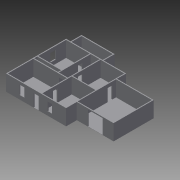
# Autodesk Inventor part: 305 Manning
Saved by Autodesk Inventor 2013 SP2 (Build 170200200, 200)
## iProperties
Created: 2014-06-03
Part Number: 305 Manning
Material: Generic
Document SubType Name: Modeling
Designer: jmw3
Density: 1 g/cm^3
Author: jmw3
Autodesk Inventor part; units mm, degrees
ref_plane "YZ Plane" through (0, 0, 0) normal (1, 0, 0) x (0, 1, 0)
ref_plane "XZ Plane" through (0, 0, 0) normal (0, 1, 0) x (-1, 0, 0)
ref_plane "XY Plane" through (0, 0, 0) normal (0, 0, 1) x (1, 0, 0)
sketch "Sketch1" plane through (0, 0, 0) normal (0, 1, 0) x (-1, 0, 0)
  line L0 (4978.4, 4978.4) -> (4978.4, -4978.4)
  line L1 (8188.96, 0) -> (-14284.96, 0) projected
  line L2 (0, -9164.32) -> (0, 7335.52) projected
  line L3 (-4978.4, -3454.4) -> (-11074.4, -3454.4)
  line L4 (-11074.4, -3454.4) -> (-11074.4, 3200.4)
  line L5 (-4978.4, -3302) -> (-10922, -3302)
  line L6 (-10922, -3302) -> (-10922, 3048)
  line L7 (4089.4, -4978.4) -> (-1092.2, -4978.4)
  line L8 (-1244.6, -4978.4) -> (-1244.6, -6807.2)
  line L9 (-1244.6, -6807.2) -> (4241.8, -6807.2)
  line L10 (4241.8, -6807.2) -> (4241.8, -4978.4)
  line L11 (4089.4, -6654.8) -> (-1092.2, -6654.8)
  line L12 (-1092.2, -6654.8) -> (-1092.2, -4978.4)
  line L13 (-1092.2, -4978.4) -> (4089.4, -4978.4)
  line L14 (4089.4, -4978.4) -> (4089.4, -6654.8)
  line L15 (-1244.6, -4978.4) -> (-4978.4, -4978.4)
  line L16 (4978.4, -4978.4) -> (4241.8, -4978.4)
  line L17 (4089.4, -4978.4) -> (-1092.2, -4978.4)
  line L18 (-4978.4, -4978.4) -> (-4978.4, -3454.4)
  line L19 (-4978.4, 3200.4) -> (-4978.4, 4978.4)
  line L20 (-6807.2, 3048) -> (-6807.2, 3200.4)
  line L21 (-9245.6, 3048) -> (-9245.6, 3200.4)
  line L22 (-10922, 3048) -> (-9245.6, 3048)
  line L23 (-6807.2, 3048) -> (-4978.4, 3048)
  line L24 (-11074.4, 3200.4) -> (-9245.6, 3200.4)
  line L25 (-6807.2, 3200.4) -> (-4978.4, 3200.4)
  line L26 (-406.4, 4826) -> (-406.4, 4978.4)
  line L27 (406.4, 4826) -> (406.4, 4978.4)
  line L28 (-4978.4, 4978.4) -> (-406.4, 4978.4)
  line L29 (406.4, 4978.4) -> (4978.4, 4978.4)
  line L30 (406.4, 4826) -> (4826, 4826)
  line L31 (4826, -203.2) -> (889, -203.2)
  line L32 (4826, -50.8) -> (889, -50.8)
  line L33 (-4826, -203.2) -> (-889, -203.2)
  line L34 (-4826, -50.8) -> (-889, -50.8)
  line L35 (-4826, -1905) -> (-4978.4, -1905)
  line L36 (-4826, -2692.4) -> (-4978.4, -2692.4)
  line L37 (-4978.4, 3048) -> (-4978.4, -1905)
  line L38 (-4978.4, -2692.4) -> (-4978.4, -3302)
  line L39 (-4978.4, 3048) -> (-4978.4, -1905)
  line L40 (-4978.4, -2692.4) -> (-4978.4, -3302)
  line L41 (-4826, -4826) -> (-4826, -2692.4)
  line L42 (-4978.4, -3302) -> (-4978.4, -2692.4)
  line L43 (-4978.4, -1905) -> (-4978.4, 3048)
  line L44 (-4826, -1905) -> (-4826, -203.2)
  line L45 (-4826, -50.8) -> (-4826, 4826)
  line L46 (-4826, 4826) -> (-889, 4826)
  line L47 (-736.6, 4826) -> (-406.4, 4826)
  line L48 (4826, -203.2) -> (4826, -4826)
  line L49 (4826, -4826) -> (889, -4826)
  line L50 (736.6, -4826) -> (-736.6, -4826)
  line L51 (-889, -4826) -> (-4826, -4826)
  line L52 (889, -2692.4) -> (736.6, -2692.4)
  line L53 (889, -3454.4) -> (736.6, -3454.4)
  line L54 (-736.6, -1016) -> (-889, -1016)
  line L55 (-736.6, -1828.8) -> (-889, -1828.8)
  line L56 (-254, 457.2) -> (-254, 609.6)
  line L57 (558.8, 609.6) -> (4826, 609.6)
  line L58 (736.6, -50.8) -> (736.6, 457.2)
  line L59 (889, -50.8) -> (889, 457.2)
  line L60 (-736.6, 3048) -> (-889, 3048)
  line L61 (-736.6, 2286) -> (-889, 2286)
  line L62 (558.8, 457.2) -> (558.8, 609.6)
  line L63 (-254, 609.6) -> (-736.6, 609.6)
  line L64 (-736.6, 457.2) -> (-254, 457.2)
  line L65 (-736.6, -50.8) -> (-736.6, 457.2)
  line L66 (4826, 457.2) -> (889, 457.2)
  line L67 (736.6, 457.2) -> (558.8, 457.2)
  line L68 (-736.6, 609.6) -> (-736.6, 2286)
  line L69 (-736.6, 3048) -> (-736.6, 4826)
  line L70 (-889, -50.8) -> (-889, 2286)
  line L71 (-889, 3048) -> (-889, 4826)
  line L72 (-736.6, -50.8) -> (-736.6, -1016)
  line L73 (-736.6, -1828.8) -> (-736.6, -4826)
  line L74 (-889, -203.2) -> (-889, -1016)
  line L75 (-889, -1828.8) -> (-889, -4826)
  line L76 (736.6, -50.8) -> (736.6, -2692.4)
  line L77 (736.6, -3454.4) -> (736.6, -4826)
  line L78 (889, -203.2) -> (889, -2692.4)
  line L79 (889, -3454.4) -> (889, -4826)
  line L80 (4826, 4826) -> (4826, 609.6)
  line L81 (4826, 457.2) -> (4826, -50.8)
  point P0 (0, 0)
  dimension "d8" = 152.4
  dimension "d9" = 152.4
  dimension "d12" = 736.6
  dimension "d14" = 152.4
  dimension "d15" = 152.4
  dimension "d16" = 152.4
  dimension "d17" = 1828.8
  dimension "d19" = 1524
  dimension "d22" = 9956.8
  dimension "d23" = 3733.8
  dimension "d24" = 1828.8
  dimension "d25" = 1828.8
  dimension "d26" = 6654.8
  dimension "d27" = 152.4
  dimension "d28" = 4572
  dimension "d29" = 812.8
  dimension "d30" = 9956.8
  dimension "d32" = 152.4
  dimension "d35" = 1701.8
  dimension "d36" = 2489.2
  dimension "d38" = 5486.4
  dimension "d40" = 152.4
  dimension "d41" = 4622.8
  dimension "d42" = 152.4
  dimension "d43" = 6096
  dimension "d44" = 2489.2
  dimension "d45" = 3251.2
  dimension "d48" = 812.8
  dimension "d49" = 812.8
  dimension "d52" = 1778
  dimension "d53" = 2540
  dimension "d57" = 812.8
  dimension "d59" = 152.4
  dimension "d60" = 152.4
  dimension "d61" = 152.4
  dimension "d62" = 5283.2
  dimension "d63" = 3937
  dimension "d64" = 4267.2
  dimension "d65" = 152.4
  constraints: 160 end point, 62 perpendicular, 49 parallel, 27 collinear, 12 horizontal, 6 symmetric about line, 2 other
  measures "d8" distance between parallel lines of L3 L5
  measures "d9" distance between parallel lines of L4 L6
  measures "d12" distance between parallel lines of L0 L10
  measures "d14" distance between parallel lines of L9 L11
  measures "d15" distance between parallel lines of L10 L14
  measures "d16" distance between parallel lines of L8 L12
  measures "d17" distance between parallel lines of L16 L9
  measures "d19" distance between parallel lines of L3 L15
  measures "d22" distance between parallel lines of L19 L0
  measures "d23" distance between parallel lines of L18 L8
  measures "d24" distance between parallel lines of L20 L19
  measures "d25" distance between parallel lines of L4 L21
  measures "d26" distance between parallel lines of L3 L24
  measures "d27" distance between parallel lines of L24 L22
  measures "d28" distance between parallel lines of L19 L26
  measures "d29" distance between parallel lines of L26 L27
  measures "d30" distance between parallel lines of L29 L7
  measures "d32" distance between parallel lines of L32 L31
  measures "d35" distance between parallel lines of L35 L33
  measures "d36" distance between parallel lines of L33 L36
  measures "d38" distance between parallel lines of L8 L10
  measures "d40" distance between parallel lines of L16 L49
  measures "d41" distance between parallel lines of L49 L31
  measures "d42" distance between parallel lines of L29 L30
  measures "d43" distance between parallel lines of L19 L4
  measures "d44" distance between parallel lines of L31 L52
  measures "d45" distance between parallel lines of L31 L53
  measures "d48" distance between parallel lines of L55 L54
  measures "d49" distance between parallel lines of L33 L54
  measures "d52" distance from line of L46 L60.end
  measures "d53" distance between parallel lines of L46 L61
  measures "d57" distance between parallel lines of L62 L56
  measures "d59" distance between parallel lines of L77 L79
  measures "d60" distance between parallel lines of L0 L48
  measures "d61" distance between parallel lines of L57 L66
  measures "d62" distance between parallel lines of L50 L67
  measures "d63" distance between parallel lines of L48 L79
  measures "d64" distance between parallel lines of L80 L62
  measures "d65" distance between parallel lines of L71 L69
extrude "Extrusion1" add sketch "Sketch1" along normal blind 2590.8 contours L0 L1 L81 L66 L59 L58 L67 L62 L57 L80 L30 L27 L29 | L0 L16 L10 L9 L2 L11 L14 L7 L50 L77 L53 L79 L49 L48 L31 L78 L52 L76 L58 L1 L59 L32 L81 | L9 L8 L15 L18 L3 L4 L1 L6 L5 L38 L36 L41 L51 L75 L55 L73 L50 L2 L7 L12 L11 | L65 L72 L54 L74 L33 L44 L35 L37 L1 L45 L34 L70 | L1 L70 L61 L68 L63 L56 L64 L65 | L1 L37 L23 L20 L25 L19 L28 L26 L47 L69 L60 L71 L46 L45 | L1 L4 L24 L21 L22 L6
sketch "Sketch2" plane through (0, 0, 0) normal (0, -1, 0) x (1, 0, 0)
  line L0 (-4978.4, -4978.4) -> (-4978.4, 4978.4) projected
  line L1 (-4241.8, -4978.4) -> (-4978.4, -4978.4) projected
  line L2 (-4241.8, -6807.2) -> (-4241.8, -4978.4) projected
  line L3 (1244.6, -6807.2) -> (-4241.8, -6807.2) projected
  line L4 (1244.6, -4978.4) -> (1244.6, -6807.2) projected
  line L5 (4978.4, -4978.4) -> (1244.6, -4978.4) projected
  line L6 (4978.4, -3454.4) -> (4978.4, -4978.4) projected
  line L7 (11074.4, -3454.4) -> (4978.4, -3454.4) projected
  line L8 (11074.4, 3200.4) -> (11074.4, -3454.4) projected
  line L9 (9245.6, 3200.4) -> (11074.4, 3200.4) projected
  line L10 (9245.6, 3048) -> (9245.6, 3200.4) projected
  line L11 (10922, 3048) -> (9245.6, 3048) projected
  line L12 (10922, -3302) -> (10922, 3048) projected
  line L13 (4978.4, -3302) -> (10922, -3302) projected
  line L14 (4978.4, -2692.4) -> (4978.4, -3302) projected
  line L15 (4826, -2692.4) -> (4978.4, -2692.4) projected
  line L16 (4826, -4826) -> (4826, -2692.4) projected
  line L17 (889, -4826) -> (4826, -4826) projected
  line L18 (889, -1828.8) -> (889, -4826) projected
  line L19 (736.6, -1828.8) -> (889, -1828.8) projected
  line L20 (736.6, -4826) -> (736.6, -1828.8) projected
  line L21 (-736.6, -4826) -> (736.6, -4826) projected
  line L22 (-736.6, -3454.4) -> (-736.6, -4826) projected
  line L23 (-889, -3454.4) -> (-736.6, -3454.4) projected
  line L24 (-889, -4826) -> (-889, -3454.4) projected
  line L25 (-4826, -4826) -> (-889, -4826) projected
  line L26 (-4826, -203.2) -> (-4826, -4826) projected
  line L27 (-889, -203.2) -> (-4826, -203.2) projected
  line L28 (-889, -2692.4) -> (-889, -203.2) projected
  line L29 (-736.6, -2692.4) -> (-889, -2692.4) projected
  line L30 (-736.6, 457.2) -> (-736.6, -2692.4) projected
  line L31 (-558.8, 457.2) -> (-736.6, 457.2) projected
  line L32 (-558.8, 609.6) -> (-558.8, 457.2) projected
  line L33 (-4826, 609.6) -> (-558.8, 609.6) projected
  line L34 (-4826, 4826) -> (-4826, 609.6) projected
  line L35 (-406.4, 4826) -> (-4826, 4826) projected
  line L36 (-406.4, 4978.4) -> (-406.4, 4826) projected
  line L37 (-4978.4, 4978.4) -> (-406.4, 4978.4) projected
  line L38 (4978.4, 4978.4) -> (4978.4, 3200.4) projected
  line L39 (406.4, 4978.4) -> (4978.4, 4978.4) projected
  line L40 (406.4, 4826) -> (406.4, 4978.4) projected
  line L41 (736.6, 4826) -> (406.4, 4826) projected
  line L42 (736.6, 3048) -> (736.6, 4826) projected
  line L43 (889, 3048) -> (736.6, 3048) projected
  line L44 (889, 4826) -> (889, 3048) projected
  line L45 (4826, 4826) -> (889, 4826) projected
  line L46 (4826, -50.8) -> (4826, 4826) projected
  line L47 (889, -50.8) -> (4826, -50.8) projected
  line L48 (889, 2286) -> (889, -50.8) projected
  line L49 (736.6, 2286) -> (889, 2286) projected
  line L50 (736.6, 609.6) -> (736.6, 2286) projected
  line L51 (254, 609.6) -> (736.6, 609.6) projected
  line L52 (254, 457.2) -> (254, 609.6) projected
  line L53 (736.6, 457.2) -> (254, 457.2) projected
  line L54 (736.6, -1016) -> (736.6, 457.2) projected
  line L55 (889, -1016) -> (736.6, -1016) projected
  line L56 (889, -203.2) -> (889, -1016) projected
  line L57 (4826, -203.2) -> (889, -203.2) projected
  line L58 (4826, -1905) -> (4826, -203.2) projected
  line L59 (4978.4, -1905) -> (4826, -1905) projected
  line L60 (4978.4, 3048) -> (4978.4, -1905) projected
  line L61 (6807.2, 3048) -> (4978.4, 3048) projected
  line L62 (6807.2, 3200.4) -> (6807.2, 3048) projected
  line L63 (4978.4, 3200.4) -> (6807.2, 3200.4) projected
  line L64 (-4978.4, 4978.4) -> (4978.4, 4978.4)
  line L65 (4978.4, 4978.4) -> (4978.4, -4978.4)
  line L66 (4978.4, -4978.4) -> (-4978.4, -4978.4)
  line L67 (-4978.4, -4978.4) -> (-4978.4, 4978.4)
  line L68 (-4241.8, -4978.4) -> (1244.6, -4978.4)
  line L69 (1244.6, -4978.4) -> (1244.6, -6807.2)
  line L70 (1244.6, -6807.2) -> (-4241.8, -6807.2)
  line L71 (-4241.8, -6807.2) -> (-4241.8, -4978.4)
  line L72 (11074.4, 3200.4) -> (4978.4, 3200.4)
  line L73 (4978.4, 3200.4) -> (4978.4, -3454.4)
  line L74 (4978.4, -3454.4) -> (11074.4, -3454.4)
  line L75 (11074.4, -3454.4) -> (11074.4, 3200.4)
  point P0 (0, 0)
  constraints: 24 end point, 6 parallel, 3 horizontal, 3 perpendicular
extrude "Extrusion2" add sketch "Sketch2" along normal blind 25.4
sketch "Sketch3" plane through (0, 2590.8, 0) normal (0, 1, 0) x (1, 0, 0)
  line L0 (6807.2, -3200.4) -> (6807.2, -3048) projected
  line L1 (9245.6, -3200.4) -> (6807.2, -3200.4) projected
  line L2 (9245.6, -3048) -> (9245.6, -3200.4) projected
  line L3 (10922, -3048) -> (9245.6, -3048) projected
  line L4 (10922, 3302) -> (10922, -3048) projected
  line L5 (4978.4, 3302) -> (10922, 3302) projected
  line L6 (4978.4, 2692.4) -> (4978.4, 3302) projected
  line L7 (4826, 2692.4) -> (4978.4, 2692.4) projected
  line L8 (4826, 4826) -> (4826, 2692.4) projected
  line L9 (889, 4826) -> (4826, 4826) projected
  line L10 (889, 1828.8) -> (889, 4826) projected
  line L11 (736.6, 1828.8) -> (889, 1828.8) projected
  line L12 (736.6, 4826) -> (736.6, 1828.8) projected
  line L13 (-736.6, 4826) -> (736.6, 4826) projected
  line L14 (-736.6, 3454.4) -> (-736.6, 4826) projected
  line L15 (-889, 3454.4) -> (-736.6, 3454.4) projected
  line L16 (-889, 4826) -> (-889, 3454.4) projected
  line L17 (-4826, 4826) -> (-889, 4826) projected
  line L18 (-4826, 203.2) -> (-4826, 4826) projected
  line L19 (-889, 203.2) -> (-4826, 203.2) projected
  line L20 (-889, 2692.4) -> (-889, 203.2) projected
  line L21 (-736.6, 2692.4) -> (-889, 2692.4) projected
  line L22 (-736.6, -457.2) -> (-736.6, 2692.4) projected
  line L23 (-558.8, -457.2) -> (-736.6, -457.2) projected
  line L24 (-558.8, -609.6) -> (-558.8, -457.2) projected
  line L25 (-4826, -609.6) -> (-558.8, -609.6) projected
  line L26 (-4826, -4826) -> (-4826, -609.6) projected
  line L27 (-406.4, -4826) -> (-4826, -4826) projected
  line L28 (-406.4, -4978.4) -> (-406.4, -4826) projected
  line L29 (406.4, -4978.4) -> (-406.4, -4978.4) projected
  line L30 (406.4, -4826) -> (406.4, -4978.4) projected
  line L31 (736.6, -4826) -> (406.4, -4826) projected
  line L32 (736.6, -3048) -> (736.6, -4826) projected
  line L33 (889, -3048) -> (736.6, -3048) projected
  line L34 (889, -4826) -> (889, -3048) projected
  line L35 (4826, -4826) -> (889, -4826) projected
  line L36 (4826, 50.8) -> (4826, -4826) projected
  line L37 (889, 50.8) -> (4826, 50.8) projected
  line L38 (889, -2286) -> (889, 50.8) projected
  line L39 (736.6, -2286) -> (889, -2286) projected
  line L40 (736.6, -609.6) -> (736.6, -2286) projected
  line L41 (254, -609.6) -> (736.6, -609.6) projected
  line L42 (254, -457.2) -> (254, -609.6) projected
  line L43 (736.6, -457.2) -> (254, -457.2) projected
  line L44 (736.6, 1016) -> (736.6, -457.2) projected
  line L45 (889, 1016) -> (736.6, 1016) projected
  line L46 (889, 203.2) -> (889, 1016) projected
  line L47 (4826, 203.2) -> (889, 203.2) projected
  line L48 (4826, 1905) -> (4826, 203.2) projected
  line L49 (4978.4, 1905) -> (4826, 1905) projected
  line L50 (4978.4, -3048) -> (4978.4, 1905) projected
  line L51 (6807.2, -3048) -> (4978.4, -3048) projected
  line L52 (-406.4, -4826) -> (406.4, -4826)
  line L53 (406.4, -4826) -> (406.4, -4978.4)
  line L54 (406.4, -4978.4) -> (-406.4, -4978.4)
  line L55 (-406.4, -4978.4) -> (-406.4, -4826)
  line L56 (736.6, -2286) -> (889, -2286)
  line L57 (889, -2286) -> (889, -3048)
  line L58 (889, -3048) -> (736.6, -3048)
  line L59 (736.6, -3048) -> (736.6, -2286)
  line L60 (-558.8, -457.2) -> (254, -457.2)
  line L61 (254, -457.2) -> (254, -609.6)
  line L62 (254, -609.6) -> (-558.8, -609.6)
  line L63 (-558.8, -609.6) -> (-558.8, -457.2)
  line L64 (736.6, 1828.8) -> (889, 1828.8)
  line L65 (889, 1828.8) -> (889, 1016)
  line L66 (889, 1016) -> (736.6, 1016)
  line L67 (736.6, 1016) -> (736.6, 1828.8)
  line L68 (-889, 3454.4) -> (-736.6, 3454.4)
  line L69 (-736.6, 3454.4) -> (-736.6, 2692.4)
  line L70 (-736.6, 2692.4) -> (-889, 2692.4)
  line L71 (-889, 2692.4) -> (-889, 3454.4)
  line L72 (4826, 2692.4) -> (4978.4, 2692.4)
  line L73 (4978.4, 2692.4) -> (4978.4, 1905)
  line L74 (4978.4, 1905) -> (4826, 1905)
  line L75 (4826, 1905) -> (4826, 2692.4)
  line L76 (6807.2, -3048) -> (9245.6, -3048)
  line L77 (9245.6, -3048) -> (9245.6, -3200.4)
  line L78 (9245.6, -3200.4) -> (6807.2, -3200.4)
  line L79 (6807.2, -3200.4) -> (6807.2, -3048)
  point P0 (0, 0)
  constraints: 56 end point, 14 parallel, 7 horizontal, 7 perpendicular
extrude "Extrusion3" add sketch "Sketch3" against normal blind 558.8 contours L49 L75 L7 L73 | L45 L67 L11 L65 | L42 L62 L24 L60
extrude "Extrusion4" add sketch "Sketch3" against normal blind 533.4 contours L39 L57 L33 L59
extrude "Extrusion5" add sketch "Sketch3" against normal blind 584.2 contours L69 L21 L71 L15
extrude "Extrusion6" add sketch "Sketch3" against normal blind 177.8 contours L0 L76 L2 L1
extrude "Extrusion7" add sketch "Sketch3" against normal blind 533.4 contours L52 L30 L29 L28
sketch "Sketch4" plane through (-4978.4, 2590.8, 4978.4) normal (0, 0, 1) x (1, 0, 0)
  line L0 (0, 0) -> (9956.8, 0) projected
  line L1 (0, -2616.2) -> (0, 0) projected
  line L2 (9956.8, 0) -> (9956.8, -2616.2) projected
  line L3 (4572, -2590.8) -> (152.4, -2590.8) projected
  line L4 (9804.4, -2590.8) -> (5867.4, -2590.8) projected
  line L5 (2235.2, -482.6) -> (3048, -482.6)
  line L6 (3048, -482.6) -> (3048, -1955.8)
  line L7 (3048, -1955.8) -> (2235.2, -1955.8)
  line L8 (2235.2, -1955.8) -> (2235.2, -482.6)
  line L9 (6908.8, -584.2) -> (7645.4, -584.2)
  line L10 (7645.4, -584.2) -> (7645.4, -1955.8)
  line L11 (7645.4, -1955.8) -> (6908.8, -1955.8)
  line L12 (6908.8, -1955.8) -> (6908.8, -584.2)
  point P0 (4978.4, -2590.8)
  dimension "d80" = 482.6
  dimension "d81" = 635
  dimension "d82" = 2235.2
  dimension "d83" = 812.8
  dimension "d84" = 635
  dimension "d85" = 584.2
  dimension "d86" = 2311.4
  dimension "d87" = 736.6
  constraints: 16 end point, 4 parallel, 2 horizontal, 2 perpendicular
  measures "d80" distance between parallel lines of L0 L5
  measures "d81" distance between parallel lines of L3 L7
  measures "d82" distance between parallel lines of L1 L8
  measures "d83" distance between parallel lines of L8 L6
  measures "d84" distance between parallel lines of L4 L11
  measures "d85" distance between parallel lines of L0 L9
  measures "d86" distance between parallel lines of L2 L10
  measures "d87" distance between parallel lines of L12 L10
extrude "Extrusion8" cut sketch "Sketch4" against normal up to surface (152.4 mm away)
sketch "Sketch6" plane through (-4826, 2590.8, -203.2) normal (1, 0, 0) x (0, 0, -1)
  line L0 (0, -2590.8) -> (4622.8, -2590.8) projected
  line L1 (0, -2590.8) -> (0, 0) projected
  line L2 (2006.6, -584.2) -> (2921, -584.2)
  line L3 (2921, -584.2) -> (2921, -1955.8)
  line L4 (2921, -1955.8) -> (2006.6, -1955.8)
  line L5 (2006.6, -1955.8) -> (2006.6, -584.2)
  point P0 (-203.2, -2590.8)
  dimension "d97" = 914.4
  dimension "d98" = 1371.6
  dimension "d99" = 635
  dimension "d100" = 2006.6
  constraints: 8 end point, 2 parallel, 1 horizontal, 1 perpendicular
  measures "d97" distance between parallel lines of L3 L5
  measures "d98" distance between parallel lines of L2 L4
  measures "d99" distance between parallel lines of L0 L4
  measures "d100" distance between parallel lines of L1 L5
extrude "Extrusion10" cut sketch "Sketch6" against normal up to surface (152.4 mm away)
body "Solid1"
